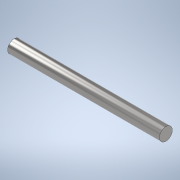
# Autodesk Inventor part: Eixo Compressor
Saved by Autodesk Inventor 2022 (Build 260153000, 153)
## iProperties
Created: 2023-07-21
Part Number: Eixo Compressor
Material: Steel, Carbon
Document SubType Name: Modeling
Designer: SENAI
Mass: 213.889 g
Surface Area: 80.9274 cm^2
Volume: 27.247 cm^3
Density: 7.85 g/cm^3
Appearance: Semi-Polished
Author: SENAI
Autodesk Inventor part; units mm, degrees
ref_plane "YZ Plane" through (0, 0, 0) normal (1, 0, 0) x (0, 1, 0)
ref_plane "XZ Plane" through (0, 0, 0) normal (0, 1, 0) x (-1, 0, 0)
ref_plane "XY Plane" through (0, 0, 0) normal (0, 0, 1) x (1, 0, 0)
sketch "Sketch1" plane through (0, 0, 0) normal (0, 0, 1) x (1, 0, 0)
  line L0 (0, 0) -> (177, 0)
  line L1 (0, 7.5) -> (177, 7.5)
  line L2 (0, 7.5) -> (0, 0)
  line L3 (177, 7.5) -> (177, 0)
  dimension "d0" = 177
  dimension "d2" = 15
  constraints: 8 end point, 2 horizontal, 2 vertical
  measures "d0" distance of L0.start L0.end
  measures "d2" diameter of L1 L0
revolve "Revolution1" add sketch "Sketch1" angle 360 about axis through (0, 0, 0) along (1, 0, 0)
body "Solid1"
